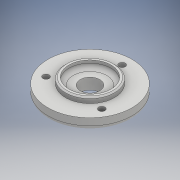
# Autodesk Inventor part: 2강2
Saved by Autodesk Inventor 2018.3 (Build 223284000, 284)
## iProperties
Created: 2019-10-09
Part Number: 2강2
Material: 일반
Document SubType Name: Modeling
Designer: MyTool
Density: 1 g/cm^3
Appearance: 기본값
Author: MyTool
Autodesk Inventor part; units mm, degrees
ref_plane "YZ Plane" through (0, 0, 0) normal (1, 0, 0) x (0, 1, 0)
ref_plane "XZ Plane" through (0, 0, 0) normal (0, 1, 0) x (-1, 0, 0)
ref_plane "XY Plane" through (0, 0, 0) normal (0, 0, 1) x (1, 0, 0)
sketch "스케치1" plane through (0, 0, 0) normal (0, 0, 1) x (1, 0, 0)
  circle A0 centre (0, 0) radius 30
  dimension "d0" = 60
  constraints: 1 centre point, 1 coincident
  measures "d0" diameter of A0
extrude "돌출1" add sketch "스케치1" along normal blind 8
sketch "스케치2" plane through (0, 0, 8) normal (0, 0, 1) x (1, 0, 0)
  circle A0 centre (0, 0) radius 17.5
  dimension "d3" = 35
  constraints: 1 centre point, 1 coincident
  measures "d3" diameter of A0
extrude "돌출2" add sketch "스케치2" along normal blind 4
sketch "스케치3" plane through (0, 0, 0) normal (0, 0, -1) x (-1, 0, 0)
  circle A0 centre (0, 0) radius 16
  dimension "d6" = 32
  constraints: 1 centre point, 1 coincident
  measures "d6" diameter of A0
extrude "돌출3" add sketch "스케치3" along normal blind 4
sketch "스케치4" plane through (0, 0, 12) normal (0, 0, 1) x (1, 0, 0)
  circle A0 centre (0, 0) radius 15
  dimension "d9" = 30
  constraints: 1 centre point, 1 coincident
  measures "d9" diameter of A0
extrude "돌출4" cut sketch "스케치4" against normal blind 5
sketch "스케치5" plane through (0, 0, 7) normal (0, 0, 1) x (1, 0, 0)
  circle A0 centre (0, 0) radius 7
  dimension "d12" = 14
  constraints: 1 centre point, 1 coincident
  measures "d12" diameter of A0
extrude "돌출5" cut sketch "스케치5" against normal blind 8
sketch "스케치6" plane through (0, 0, -1) normal (0, 0, 1) x (1, 0, 0)
  circle A0 centre (0, 0) radius 12.5
  dimension "d15" = 25
  constraints: 1 centre point, 1 coincident
  measures "d15" diameter of A0
extrude "돌출6" cut sketch "스케치6" against normal up to next
sketch "스케치7" plane through (0, 0, 0) normal (0, 0, -1) x (-1, 0, 0)
  circle A0 centre (0, 23) radius 2.25
  point P0 (0, 0)
  dimension "d18" = 4.5
  dimension "d19" = 23
  constraints: 1 centre point
  measures "d18" diameter of A0
  measures "d19" distance of point (0, 0) A0.centre
hole "구멍1" at (0, 23, 0) direction (0, 0, 1) diameter 4.5 end through all counterbore diameter 8 counterbore depth 4.4
pattern_circular "원형 패턴1" count 3 over 360 about axis through (0, 0, 0) along (0, 0, 1) of "구멍1"
chamfer "모따기1" distance 0.4 angle 30 1 edges at (-12.5, 0, -4) measured on face at (12.4595, -1.0058, -3)
fillet "모깎기1" radius 0.5 1 edges at (-12.5, 0, -1)
chamfer "모따기2" distance 1 angle 45 1 edges at (-17.5, 0, 12)
fillet "모깎기2" radius 3 4 edges at (-30, 0, 0) (16, 0, 0) (16, 0, -4) (-15, 0, 7)
